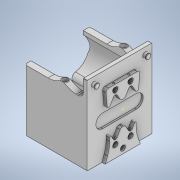
# Autodesk Inventor part: akkum_base2
Saved by Autodesk Inventor 2022 (Build 260153000, 153)
## iProperties
Created: 2024-07-26
Part Number: akkum_base2
Material: Типовые
Document SubType Name: Modeling
Designer: Капустяник Андрей
Density: 1 g/cm^3
Appearance: По умолчанию
Author: Капустяник Андрей
Autodesk Inventor part; units mm, degrees
ref_plane "YZ Plane" through (0, 0, 0) normal (1, 0, 0) x (0, 1, 0)
ref_plane "XZ Plane" through (0, 0, 0) normal (0, 1, 0) x (-1, 0, 0)
ref_plane "XY Plane" through (0, 0, 0) normal (0, 0, 1) x (1, 0, 0)
sketch "Эскиз1" plane through (0, 0, 0) normal (1, 0, 0) x (0, 1, 0)
  circle A0 centre (3.5, 9.3) radius 9.5 projected
  circle A1 centre (3.5, -9.3) radius 9.5 projected
  circle A2 centre (-12.6081, 0) radius 9.5 projected
  line L0 (-24, -20) -> (24, -20) projected
  line L1 (-24, 20) -> (-24, -20) projected
  line L2 (24, 20) -> (-24, 20) projected
  line L3 (13, -19) -> (13, 19) projected
  line L4 (24, -20) -> (24, 20) projected
  line L5 (-23.5, 19.5) -> (-23.5, -19.5)
  line L6 (-23.5, -19.5) -> (23.5, -19.5)
  line L7 (23.5, -19.5) -> (23.5, 19.5)
  line L8 (23.5, 19.5) -> (-23.5, 19.5)
  line L9 (-23.2, 19.2) -> (-23.2, -19.2)
  line L10 (-23.2, -19.2) -> (23.2, -19.2)
  line L11 (23.2, -19.2) -> (23.2, 19.2)
  line L12 (23.2, 19.2) -> (-23.2, 19.2)
  line L13 (13, 19.2) -> (13, -19.2)
  circle A3 centre (-8.3458, 11.2175) radius 2.5
  circle A4 centre (-8.3458, -11.2175) radius 2.5
  circle A5 centre (11.0835, 0) radius 2.5
  point P0 (0, 0)
  point P1 (13, 9.3)
  point P2 (13, -9.3)
  point P3 (-5.5236, -6.3293)
  point P4 (-5.5236, 6.3293)
  point P5 (5.4391, 0)
  point P6 (-5.8779, -10.818)
  point P7 (-9.2338, -8.8805)
  point P8 (-9.2338, 8.8805)
  point P9 (-5.8779, 10.818)
  point P10 (9.5036, 1.9375)
  point P11 (9.5036, -1.9375)
  dimension "d2" = 0.5
  dimension "d3" = 0.3
  dimension "d4" = 5
  dimension "d5" = 5
  dimension "d6" = 5
  constraints: 18 end point, 6 tangent, 3 centre point, 3 point on line, 1 collinear, 6 other
  measures "d2" distance between parallel lines of L2 L8
  measures "d3" distance between parallel lines of L8 L12
  measures "d4" diameter of A3
  measures "d5" diameter of A4
  measures "d6" diameter of A5
extrude "Выдавливание1" add sketch "Эскиз1" along normal blind 34.5 contours L3 A5 A0 | A0 A3 A2 A4 A1 L3 L13 L10 L9 L12 | A3 | A5 L3 | A5 L3 A1 | A4 picked at (11.5482, -0.1832)
sketch "Эскиз2" plane through (34.5, 0, 0) normal (1, 0, 0) x (0, 0, -1)
  line L0 (19.2, -23.2) -> (19.2, 13) projected
  line L1 (19.2, 13) -> (9.3, 13) projected
  arc A0 (10.818, -5.8779) -> (9.3, 13) centre (9.3, 3.5) ccw projected
  arc A1 (10.818, -5.8779) -> (8.8805, -9.2338) centre (11.2175, -8.3458) ccw projected
  arc A2 (-8.8805, -9.2338) -> (8.8805, -9.2338) centre (0, -12.6081) ccw projected
  arc A3 (-8.8805, -9.2338) -> (-10.818, -5.8779) centre (-11.2175, -8.3458) ccw projected
  arc A4 (-9.3, 13) -> (-10.818, -5.8779) centre (-9.3, 3.5) ccw projected
  line L2 (-9.3, 13) -> (-19.2, 13) projected
  line L3 (-19.2, 13) -> (-19.2, -23.2) projected
  line L4 (-19.2, -23.2) -> (19.2, -23.2) projected
  circle A5 centre (-9.3, 3.5) radius 7.5
  circle A6 centre (9.3, 3.5) radius 7.5
  circle A7 centre (0, -12.6081) radius 7.5
  circle A8 centre (11.2175, -8.3458) radius 4.5
  circle A9 centre (-11.2175, -8.3458) radius 4.5
  arc A10 (-1.9375, 9.5036) -> (1.9375, 9.5036) centre (0, 11.0835) ccw projected
  circle A11 centre (0, 11.0835) radius 4.5
  arc A12 (-1.9375, 9.5036) -> (-9.3, 13) centre (-9.3, 3.5) ccw projected
  arc A13 (-1.9375, 9.5036) -> (1.9375, 9.5036) centre (0, 11.0835) ccw projected
  arc A14 (9.3, 13) -> (1.9375, 9.5036) centre (9.3, 3.5) ccw projected
  line L5 (9.3, 13) -> (-9.3, 13) projected
  point P0 (0, 0)
  point P1 (-9.3, 13)
  point P2 (9.3, 13)
  point P3 (-3.4875, 8.2397)
  point P4 (3.4875, 8.2397)
  point P5 (10.4985, -3.9036)
  point P6 (7.011, -9.9442)
  point P7 (-7.011, -9.9442)
  point P8 (-10.4985, -3.9036)
  dimension "d7" = 15
  dimension "d8" = 15
  dimension "d9" = 15
  constraints: 6 centre point, 6 coincident, 3 tangent
  measures "d7" diameter of A5
  measures "d8" diameter of A6
  measures "d9" diameter of A7
extrude "Выдавливание2" add sketch "Эскиз2" against normal blind 1.7 contours L4 L3 L2 A4 A9 A2 A8 A0 L1 L0 | A0 A8 A6 A11 A14 | A14 A11 L5 | A8 A2 A1 A0 | A0 A1 A2 A8 | A14 A10 A12 A11 L5 | A11 A12 A10 A14 | A12 A11 A5 A9 A4 | L5 A11 A12 | A9 A2 A3 A4 | A4 A3 A2 A9 | A2 A9 A7 A8
sketch "Эскиз3" plane through (34.5, 0, 0) normal (1, 0, 0) x (0, 0, -1)
  line L0 (-15.5, 15.5) -> (-15.5, 17.5) projected
  line L1 (15.5, 17.5) -> (15.5, 15.5) projected
  line L2 (-15.5, 15.5) -> (15.5, 15.5)
  line L3 (15.5, 15.5) -> (15.5, 2)
  line L4 (15.5, 2) -> (-15.5, 2)
  line L5 (-15.5, 2) -> (-15.5, 15.5)
  point P0 (0, 0)
  constraints: 8 end point, 2 parallel, 1 collinear, 1 horizontal, 1 perpendicular
extrude "Выдавливание3" cut sketch "Эскиз3" against normal blind 2
sketch "Эскиз4" plane through (34.5, 0, 0) normal (1, 0, 0) x (0, 0, -1)
  line L0 (15.5, 13) -> (15.5, 7.7202) projected
  arc A0 (10.4985, -3.9036) -> (15.5, 7.7202) centre (9.3, 3.5) ccw projected
  arc A1 (10.4985, -3.9036) -> (7.011, -9.9442) centre (11.2175, -8.3458) ccw projected
  arc A2 (-7.011, -9.9442) -> (7.011, -9.9442) centre (0, -12.6081) ccw projected
  arc A3 (-7.011, -9.9442) -> (-10.4985, -3.9036) centre (-11.2175, -8.3458) ccw projected
  arc A4 (-15.5, 7.7202) -> (-10.4985, -3.9036) centre (-9.3, 3.5) ccw projected
  line L1 (-15.5, 7.7202) -> (-15.5, 13) projected
  line L2 (-15.5, 13) -> (-19.2, 13) projected
  line L3 (-19.2, 13) -> (-19.2, -23.2) projected
  line L4 (-19.2, -23.2) -> (19.2, -23.2) projected
  line L5 (19.2, -23.2) -> (19.2, 13) projected
  line L6 (19.2, 13) -> (15.5, 13) projected
  line L7 (20, 24) -> (-20, 24) projected
  line L8 (-20, 24) -> (-20, -24) projected
  line L9 (20, -24) -> (20, 24) projected
  line L10 (-20, -24) -> (20, -24) projected
  line L11 (19.2, 23.2) -> (-19.2, 23.2)
  line L12 (-19.2, 23.2) -> (-19.2, -23.2)
  line L13 (-19.2, -23.2) -> (19.2, -23.2)
  line L14 (19.2, -23.2) -> (19.2, 23.2)
  point P0 (0, 0)
  point P1 (19.2, 4.494)
  dimension "d14" = 0.8
  constraints: 8 end point, 3 other
  measures "d14" distance between parallel lines of L9 L14
extrude "Выдавливание4" add sketch "Эскиз4" along normal blind 4.7 contours L6 L5 L4 L3 L2 L1 A4 A3 A2 A1 A0 L0 | L0 A0 A1 A2 A3 A4 L1 L2 L12 L11 L14 L6
sketch "Эскиз5" plane through (39.2, 0, 0) normal (1, 0, 0) x (0, 0, -1)
  line L0 (-19.5, 23.5) -> (-19.5, -23) projected
  line L1 (-20, 23.5) -> (-19.5, 23.5) projected
  line L2 (-20, -23) -> (-20, 23.5) projected
  arc A0 (-20, -23) -> (-19, -24) centre (-19, -23) ccw projected
  line L3 (-19, -23.5) -> (-19, -24) projected
  arc A1 (-19.5, -23) -> (-19, -23.5) centre (-19, -23) ccw projected
  arc A2 (19, -23.5) -> (19.5, -23) centre (19, -23) ccw projected
  line L4 (19, -24) -> (19, -23.5) projected
  arc A3 (19, -24) -> (20, -23) centre (19, -23) ccw projected
  line L5 (20, 23.5) -> (20, -23) projected
  line L6 (19.5, 23.5) -> (20, 23.5) projected
  line L7 (19.5, -23) -> (19.5, 23.5) projected
  line L8 (19.2, 23.2) -> (-19.2, 23.2) projected
  line L9 (-19.2, 23.2) -> (-19.2, -23.2) projected
  line L10 (-19.2, -23.2) -> (19.2, -23.2) projected
  line L11 (19.2, -23.2) -> (19.2, 23.2) projected
  circle A4 centre (-19, -23) radius 0.2
  circle A5 centre (19, -23) radius 0.2
  circle A6 centre (19, 23) radius 0.2
  line L12 (19.2, -23.2) -> (19.2, 23.2) projected
  circle A7 centre (-19, 23) radius 0.2
  line L13 (-19.2, 23.2) -> (-19.2, -23.2) projected
  line L14 (19.2, 23.2) -> (-19.2, 23.2) projected
  point P0 (0, 0)
  point P1 (-19, -23.2)
  point P2 (-19.2, -23)
  point P3 (19.2, -23)
  point P4 (19, -23.2)
  point P5 (19, 23.2)
  point P6 (19.2, 23)
  point P7 (-19.2, 23)
  point P8 (-19, 23.2)
  dimension "d17" = 0.4
  dimension "d18" = 0.4
  constraints: 6 tangent, 4 centre point, 2 coincident
  measures "d17" diameter of A6
  measures "d18" diameter of A7
extrude "Выдавливание5" cut sketch "Эскиз5" against normal blind 200 contours L11 A6 L8 | A7 L9 L8 | L11 L10 A5 | A4 L10 L9
sketch "Эскиз7" plane through (34.5, 0, 0) normal (-1, 0, 0) x (0, 0, 1)
  arc A0 (-19, 23.2) -> (-19.2, 23) centre (-19, 23) ccw projected
  line L0 (-19.2, 13) -> (-19.2, 23) projected
  line L1 (-19.2, 13) -> (-15.5, 13) projected
  line L2 (-15.5, 13) -> (-15.5, 7.7202) projected
  arc A1 (-15.5, 7.7202) -> (-10.4985, -3.9036) centre (-9.3, 3.5) ccw projected
  arc A2 (-7.011, -9.9442) -> (-10.4985, -3.9036) centre (-11.2175, -8.3458) ccw projected
  arc A3 (-7.011, -9.9442) -> (7.011, -9.9442) centre (0, -12.6081) ccw projected
  arc A4 (10.4985, -3.9036) -> (7.011, -9.9442) centre (11.2175, -8.3458) ccw projected
  arc A5 (10.4985, -3.9036) -> (15.5, 7.7202) centre (9.3, 3.5) ccw projected
  line L3 (15.5, 7.7202) -> (15.5, 13) projected
  line L4 (15.5, 13) -> (19.2, 13) projected
  line L5 (19.2, 23) -> (19.2, 13) projected
  arc A6 (19.2, 23) -> (19, 23.2) centre (19, 23) ccw projected
  line L6 (-19, 23.2) -> (19, 23.2) projected
  line L7 (15.5, 13) -> (19.2, 13) projected
  line L8 (-15.5, 13) -> (15.5, 13)
  point P0 (0, 0)
  constraints: 2 end point, 1 collinear
extrude "Выдавливание6" cut sketch "Эскиз7" against normal blind 0.5 contours L6 A6 L5 L4 L8 L1 L0 A0
sketch "Эскиз11" plane through (0, 0, 0) normal (-1, 0, 0) x (0, 0, 1)
  line L0 (15.5, 13) -> (-15.5, 13) projected
  line L1 (-15.5, 13) -> (-15.5, 7.7202) projected
  arc A0 (-15.5, 7.7202) -> (-10.4985, -3.9036) centre (-9.3, 3.5) ccw projected
  arc A1 (-7.011, -9.9442) -> (-10.4985, -3.9036) centre (-11.2175, -8.3458) ccw projected
  arc A2 (-7.011, -9.9442) -> (7.011, -9.9442) centre (0, -12.6081) ccw projected
  arc A3 (10.4985, -3.9036) -> (7.011, -9.9442) centre (11.2175, -8.3458) ccw projected
  arc A4 (10.4985, -3.9036) -> (15.5, 7.7202) centre (9.3, 3.5) ccw projected
  line L2 (15.5, 7.7202) -> (15.5, 13) projected
  point P0 (0, 0)
extrude "Выдавливание8" cut sketch "Эскиз11" against normal up to surface (34.5 mm away)
sketch "Эскиз12" plane through (0, 13, 19.2) normal (0, 1, 0) x (1, 0, 0)
  arc A0 (-32.5, 38.2) -> (-34.5, 36.2) centre (-32.5, 36.2) ccw projected
  line L0 (-34.5, 36.2) -> (-34.5, 35.7) projected
  arc A1 (-34.5, 35.7) -> (-33.5, 34.7) centre (-33.5, 35.7) ccw projected
  line L1 (-33.5, 34.7) -> (-33, 34.7) projected
  arc A2 (-32.5, 34.2) -> (-33, 34.7) centre (-33, 34.2) ccw projected
  line L2 (-32.5, 34.2) -> (-32.5, 23.2) projected
  arc A3 (-33, 22.7) -> (-32.5, 23.2) centre (-33, 23.2) ccw projected
  line L3 (-33, 22.7) -> (-33.5, 22.7) projected
  arc A4 (-33.5, 22.7) -> (-34.5, 21.7) centre (-33.5, 21.7) ccw projected
  line L4 (-34.5, 21.7) -> (-34.5, 16.7) projected
  arc A5 (-34.5, 16.7) -> (-33.5, 15.7) centre (-33.5, 16.7) ccw projected
  line L5 (-33.5, 15.7) -> (-33, 15.7) projected
  arc A6 (-32.5, 15.2) -> (-33, 15.7) centre (-33, 15.2) ccw projected
  line L6 (-32.5, 15.2) -> (-32.5, 4.2) projected
  arc A7 (-33, 3.7) -> (-32.5, 4.2) centre (-33, 4.2) ccw projected
  line L7 (-33, 3.7) -> (-33.5, 3.7) projected
  arc A8 (-33.5, 3.7) -> (-34.5, 2.7) centre (-33.5, 2.7) ccw projected
  line L8 (-34.5, 2.7) -> (-34.5, 2.2) projected
  arc A9 (-34.5, 2.2) -> (-32.5, 0.2) centre (-32.5, 2.2) ccw projected
  line L9 (-32.5, 0.2) -> (-24.6, 0.2) projected
  arc A10 (32.5, 0.2) -> (34.5, 2.2) centre (32.5, 2.2) ccw projected
  line L10 (34.5, 2.2) -> (34.5, 2.7) projected
  arc A11 (34.5, 2.7) -> (33.5, 3.7) centre (33.5, 2.7) ccw projected
  line L11 (33.5, 3.7) -> (33, 3.7) projected
  arc A12 (32.5, 4.2) -> (33, 3.7) centre (33, 4.2) ccw projected
  line L12 (32.5, 4.2) -> (32.5, 15.2) projected
  arc A13 (33, 15.7) -> (32.5, 15.2) centre (33, 15.2) ccw projected
  line L13 (33, 15.7) -> (33.5, 15.7) projected
  arc A14 (33.5, 15.7) -> (34.5, 16.7) centre (33.5, 16.7) ccw projected
  line L14 (34.5, 16.7) -> (34.5, 21.7) projected
  arc A15 (34.5, 21.7) -> (33.5, 22.7) centre (33.5, 21.7) ccw projected
  line L15 (33.5, 22.7) -> (33, 22.7) projected
  arc A16 (32.5, 23.2) -> (33, 22.7) centre (33, 23.2) ccw projected
  line L16 (32.5, 23.2) -> (32.5, 34.2) projected
  arc A17 (33, 34.7) -> (32.5, 34.2) centre (33, 34.2) ccw projected
  line L17 (33, 34.7) -> (33.5, 34.7) projected
  arc A18 (33.5, 34.7) -> (34.5, 35.7) centre (33.5, 35.7) ccw projected
  line L18 (34.5, 35.7) -> (34.5, 36.2) projected
  arc A19 (34.5, 36.2) -> (32.5, 38.2) centre (32.5, 36.2) ccw projected
  line L19 (32.5, 38.2) -> (24.6, 38.2) projected
  line L20 (0, 0) -> (35, 0) projected
  line L21 (32.5, 0) -> (32.5, 3.7)
  line L22 (34.5, 3.7) -> (0, 3.7) projected
  line L23 (0, 38.4) -> (35, 38.4) projected
  line L24 (32.5, 38.4) -> (32.5, 34.7)
  line L25 (0, 34.7) -> (34.5, 34.7) projected
  line L26 (32.5, 36.55) -> (22.5, 36.55)
  line L27 (32.5, 1.85) -> (22.5, 1.85)
  circle A20 centre (22.5, 1.85) radius 1.5
  circle A21 centre (22.5, 1.85) radius 2
  circle A22 centre (22.5, 36.55) radius 1.5
  circle A23 centre (22.5, 36.55) radius 2
  arc A24 (-21.4, 1.2) -> (-20.4, 0.2) centre (-20.4, 1.2) ccw projected
  line L28 (-20.4, 0.2) -> (1.7, 0.2) projected
  arc A25 (20.4, 0.2) -> (21.4, 1.2) centre (20.4, 1.2) ccw projected
  line L29 (21.4, 1.2) -> (21.4, 1.85) projected
  arc A26 (23.6, 1.85) -> (21.4, 1.85) centre (22.5, 1.85) ccw projected
  line L30 (23.6, 1.85) -> (23.6, 1.2) projected
  arc A27 (23.6, 1.2) -> (24.6, 0.2) centre (24.6, 1.2) ccw projected
  line L31 (24.6, 0.2) -> (32.5, 0.2) projected
  arc A28 (24.6, 38.2) -> (23.6, 37.2) centre (24.6, 37.2) ccw projected
  line L32 (23.6, 37.2) -> (23.6, 36.55) projected
  arc A29 (21.4, 36.55) -> (23.6, 36.55) centre (22.5, 36.55) ccw projected
  line L33 (21.4, 36.55) -> (21.4, 37.2) projected
  arc A30 (21.4, 37.2) -> (20.4, 38.2) centre (20.4, 37.2) ccw projected
  line L34 (20.4, 38.2) -> (-20.4, 38.2) projected
  arc A31 (-20.4, 38.2) -> (-21.4, 37.2) centre (-20.4, 37.2) ccw projected
  line L35 (-21.4, 37.2) -> (-21.4, 36.55) projected
  arc A32 (-23.6, 36.55) -> (-21.4, 36.55) centre (-22.5, 36.55) ccw projected
  line L36 (-23.6, 36.55) -> (-23.6, 37.2) projected
  arc A33 (-23.6, 37.2) -> (-24.6, 38.2) centre (-24.6, 37.2) ccw projected
  line L37 (-24.6, 38.2) -> (-32.5, 38.2) projected
  arc A34 (-24.6, 0.2) -> (-23.6, 1.2) centre (-24.6, 1.2) ccw projected
  line L38 (-23.6, 1.2) -> (-23.6, 1.85) projected
  arc A35 (-21.4, 1.85) -> (-23.6, 1.85) centre (-22.5, 1.85) ccw projected
  line L39 (-21.4, 1.85) -> (-21.4, 1.2) projected
  arc A36 (1.7, 0.2) -> (2, 0.5) centre (1.7, 0.5) ccw projected
  line L40 (2, 0.5) -> (2, 0.9) projected
  arc A37 (2.3, 1.2) -> (2, 0.9) centre (2.3, 0.9) ccw projected
  line L41 (2.3, 1.2) -> (13.7, 1.2) projected
  arc A38 (14, 0.9) -> (13.7, 1.2) centre (13.7, 0.9) ccw projected
  line L42 (14, 0.9) -> (14, 0.5) projected
  arc A39 (14, 0.5) -> (14.3, 0.2) centre (14.3, 0.5) ccw projected
  line L43 (14.3, 0.2) -> (20.4, 0.2) projected
  point P0 (0, 19.2)
  point P1 (23.6303, 38.2)
  point P2 (21.3697, 38.2)
  point P3 (21.7401, 34.7)
  point P4 (23.2599, 34.7)
  point P5 (23.2599, 3.7)
  point P6 (21.7401, 3.7)
  point P7 (21.3697, 0.2)
  point P8 (23.6303, 0.2)
  point P9 (23.2599, 0)
  point P10 (21.7401, 0)
  point P11 (23.2599, 38.4)
  point P12 (21.7401, 38.4)
  point P13 (23.9331, 37.9451)
  point P14 (21.0669, 37.9451)
  point P15 (23.9331, 0.4549)
  point P16 (21.0669, 0.4549)
  dimension "d36" = 10
  dimension "d37" = 10
  dimension "d38" = 3
  dimension "d39" = 4
  dimension "d40" = 3
  dimension "d41" = 4
  constraints: 8 end point, 4 centre point, 4 coincident, 4 point on line, 2 horizontal, 2 midpoint, 2 vertical
  measures "d36" distance of L26.start L26.end
  measures "d37" distance of L27.start L27.end
  measures "d38" diameter of A20
  measures "d39" diameter of A21
  measures "d40" diameter of A22
  measures "d41" diameter of A23
extrude "Выдавливание9" add sketch "Эскиз12" along normal blind 2.3 contours A30 A22 L26 A23 L25 | A23 L23 A28 A22 A30 | A28 A23 L26 A22 | A21 L27 A20 A25 L22 | A21 A27 A20 L27 | A21 L20 A25 A20 A27
chamfer "Фаска1" distance 2.3 angle 45 4 edges at (20.5, 13, 17.35) (24.5, 13, 17.35) (20.5, 13, -17.35) (24.5, 13, -17.35)
fillet "Сопряжение1" radius 10 4 edges at (18.2001, 13, -17.35) (26.7999, 13, -17.35) (26.7999, 13, 17.35) (18.2001, 13, 17.35)
sketch "Эскиз14" plane through (0, -23.2, -19) normal (0, -1, 0) x (1, 0, 0)
  line L0 (-25, 4) -> (25, 4)
  line L1 (25, 4) -> (25, 34)
  line L2 (25, 34) -> (-25, 34)
  line L3 (-25, 34) -> (-25, 4)
  line L4 (-25, 4) -> (25, 34) construction
  line L5 (25, 4) -> (-25, 34) construction
  line L6 (14, 34) -> (2, 34)
  line L7 (2, 38.2) -> (2, 38) projected
  line L8 (2, 38.2) -> (14, 38.2)
  line L9 (14, 38.2) -> (14, 34)
  line L10 (14, 34) -> (2, 34)
  line L11 (2, 34) -> (2, 38.2)
  line L12 (14, 38) -> (14, 38.2) projected
  point P0 (0, 19)
  dimension "d51" = 30
  constraints: 22 end point, 4 parallel, 2 horizontal, 2 midpoint, 2 perpendicular, 1 collinear, 1 point on line
  measures "d51" distance of L1.end L0.end
extrude "Выдавливание11" cut sketch "Эскиз14" against normal blind 0.8 contours L3 L2 L1 L0
fillet "Сопряжение4" radius 0.15 3 edges at (12.5, -23.2, 15) (25, -23.2, 0) (12.5, -23.2, -15)
fillet "Сопряжение5" radius 3 1 edges at (35, 13, 0)
sketch "Эскиз15" plane through (39.2, 0, 0) normal (1, 0, 0) x (0, 0, -1)
  point P0 (0, 0)
sketch "Эскиз16" plane through (0, -23, -19.2) normal (0, 0, -1) x (-1, 0, 0)
  line L0 (-39.5, 46) -> (-40, 46) projected
  arc A0 (-39, 46.5) -> (-39.5, 46) centre (-39, 46) ccw projected
  line L1 (-39, 47) -> (-39, 46.5) projected
  arc A1 (-39, 47) -> (-40, 46) centre (-39, 46) ccw projected
  line L2 (-35, 46) -> (-39.2, 46) projected
  circle A2 centre (-39, 46) radius 0.2
  line L3 (-35, 46) -> (-35, 46.2) projected
  line L4 (-35, 46.2) -> (-39.2, 46.2) projected
  line L5 (-39.2, 46) -> (-39.2, 46.2) projected
  line L6 (-35, 46) -> (-39.2, 46) projected
  line L7 (0, 36) -> (-14.3263, 36) projected
  line L8 (-23.2599, 38.3) -> (-21.7401, 38.3) projected
  line L9 (-30.6737, 36) -> (-32, 36) projected
  arc A3 (-35, 39) -> (-32, 36) centre (-32, 39) ccw projected
  line L10 (-35, 39) -> (-35, 46) projected
  line L11 (-35, 46) -> (-39.2, 46) projected
  line L12 (-39.2, 0) -> (-39.2, 46) projected
  line L13 (0, 0) -> (-39.2, 0) projected
  line L14 (0, 0) -> (0, 36) projected
  line L15 (0, 0) -> (0, -0.2) projected
  line L16 (0, 0) -> (-39.2, 0) projected
  line L17 (-39.2, -0.2) -> (-39.2, 0) projected
  line L18 (0, -0.2) -> (-39.2, -0.2) projected
  line L19 (0, 0) -> (-39.2, 0) projected
  circle A4 centre (-39, 0) radius 0.2
  point P0 (0, 23)
  point P1 (-14.15, 0)
  point P2 (-39, -0.2)
  point P3 (-39, 46.2)
  constraints: 1 centre point, 1 coincident, 1 point on line, 1 tangent, 5 other
extrude "Выдавливание12" cut sketch "Эскиз16" against normal blind 50 contours L5 L4 A2 | A4 L18 L17
sketch "Эскиз17" plane through (39.2, 0, 0) normal (1, 0, 0) x (0, 0, -1)
  line L0 (-19, 23.2) -> (19, 23.2) projected
  line L1 (-19.2, 23) -> (-19.2, -23) projected
  line L2 (19.2, -23) -> (19.2, 23) projected
  arc A0 (-19.2, -23) -> (-19, -23.2) centre (-19, -23) ccw projected
  line L3 (-19, -23.2) -> (19, -23.2) projected
  arc A1 (19, -23.2) -> (19.2, -23) centre (19, -23) ccw projected
  arc A2 (19.2, 23) -> (19, 23.2) centre (19, 23) ccw projected
  arc A3 (-19, 23.2) -> (-19.2, 23) centre (-19, 23) ccw projected
  line L4 (-19.2, 23.2) -> (-15.2, 23.2)
  line L5 (19, 23.2) -> (-19, 23.2) projected
  line L6 (-19.2, 23.2) -> (-19.2, 19.2)
  line L7 (-19.2, 23) -> (-19.2, 16) projected
  line L8 (-19.2, 19.2) -> (-15.2, 19.2)
  line L9 (-15.2, 19.2) -> (-15.2, 23.2)
  circle A4 centre (-15.2, 19.2) radius 1.6
  circle A5 centre (-15.2, 19.2) radius 4
  circle A6 centre (-15.2, 19.2) radius 1.1
  line L10 (-15.2, 19.2) -> (-15.2, 15.2)
  line L11 (0, 23.2) -> (0, -23.2)
  circle A7 centre (15.2, 19.2) radius 1.1
  circle A8 centre (-15.2, 19.2) radius 4.25
  circle A9 centre (15.2, 19.2) radius 4.25
  line L12 (-15.2, 14.95) -> (15.2, 14.95)
  line L13 (-7, 12.95) -> (-6, 12.95)
  line L14 (-6, 12.95) -> (-6, -17.05)
  line L15 (-6, -17.05) -> (-7, -17.05)
  line L16 (-7, -17.05) -> (-7, 12.95)
  circle A10 centre (-10, -2.05) radius 3
  line L17 (-7, -2.05) -> (-10, -2.05)
  line L18 (7, 12.95) -> (6, 12.95)
  line L19 (6, 12.95) -> (6, -17.05)
  line L20 (6, -17.05) -> (7, -17.05)
  line L21 (7, -17.05) -> (7, 12.95)
  circle A11 centre (10, -2.05) radius 3
  line L22 (-15.2, 15.2) -> (-1.2, 15.2)
  circle A12 centre (-15.2, 19.2) radius 14.5602
  line L23 (-19.2, 19.2) -> (-19.2, -23.2)
  circle A13 centre (-15.2, 19.2) radius 42.4
  line L24 (-15.2, -23.2) -> (-20, -23.2)
  line L25 (-20, -23.2) -> (-20.5, -23.2)
  line L26 (-26.7027, -23) -> (-27.1951, -22.9132)
  line L27 (19, -24) -> (-19, -24) projected
  line L28 (-27.1951, -22.9132) -> (-25.4586, -13.0651)
  line L29 (-25.4586, -13.0651) -> (-24.9662, -13.1519)
  circle A14 centre (-15.2, 19.2) radius 33.7939
  circle A15 centre (-15.2, 19.2) radius 43.7396
  line L30 (-26.7027, -23) -> (-20, -23)
  line L31 (-20, -23) -> (-20, 23) projected
  line L32 (-25.4586, -13.0651) -> (-20, -13.0651)
  line L33 (-26.7027, -23) -> (-19.1392, 19.8946)
  line L34 (-26.4691, -21.675) -> (-18.5906, -23.0642)
  line L35 (-25.4586, -13.0651) -> (-15.2, -13.0651)
  line L36 (-15.2, -13.0651) -> (-15.2, -14.5939)
  line L37 (-15.2, 19.2) -> (-15.2, -14.5939)
  line L38 (-24.2716, -9.2127) -> (-19.2, -9.2127)
  line L39 (-24.9662, -13.1519) -> (-24.2716, -9.2127)
  line L40 (-11.2147, 18.8576) -> (-14.8281, -23.1984)
  line L41 (-11.2158, 19.5548) -> (-7.4714, -22.4897)
  circle A16 centre (-6.2798, -2.05) radius 3
  line L42 (-7, 12.95) -> (-7, 9.95)
  line L43 (-7, 9.95) -> (-6, 9.95)
  line L44 (-7, -17.05) -> (-7, -14.05)
  line L45 (-7, -14.05) -> (-6, -14.05)
  spline S0 degree 2 poles (-7, 9.95) (0.4395, -1.9931) (-7, -14.05) knots 0 0 0 1 1 1
  line L46 (-7, 9.95) -> (-8.0386, 11.6717)
  line L47 (-8.0386, 11.6717) -> (-7.1824, 12.1882)
  line L48 (-7.1824, 12.1882) -> (-6, 9.95)
  line L49 (-3.2803, -1.9976) -> (-2.2803, -1.9976)
  spline S1 degree 2 poles (-6, 9.95) (1.4395, -1.9931) (-6, -14.05) knots 0 0 0 1 1 1
  line L50 (-7, -14.05) -> (-8.0477, -15.7629)
  line L51 (-8.0477, -15.7629) -> (-7.1947, -16.2847)
  line L52 (-7.1947, -16.2847) -> (-6, -14.05)
  line L53 (-6.5, 9.95) -> (-7.6135, 11.9281)
  line L54 (-6.5, -14.05) -> (-7.6212, -16.0238)
  line L55 (-24.2716, -9.2127) -> (-20, -9.2127)
  circle A17 centre (-15.2, 19.2) radius 29.8258
  line L56 (-24.2716, -9.2127) -> (-15.2, -9.2127)
  line L57 (-15.2, -9.2127) -> (-15.2, -10.6258)
  line L58 (-14.5054, 23.1392) -> (-0.7181, 20.7082)
  point P0 (0, 0)
  dimension "d83" = 6
  dimension "d60" = 4
  dimension "d61" = 4
  dimension "d62" = 3.2
  dimension "d63" = 8
  dimension "d64" = 2.2
  dimension "d65" = 0.25
  dimension "d66" = 1
  dimension "d67" = 30
  dimension "d68" = 6
  dimension "d69" = 2
  dimension "d70" = 6
  dimension "d71" = 14
  dimension "d73" = 0.5
  dimension "d75" = 0.5
  dimension "d76" = 10
  dimension "d77" = 1
  dimension "d78" = 10
  dimension "d79" = 1.5288
  dimension "d80" = 4
  dimension "d82" = 10
  dimension "d84" = 3
  dimension "d85" = 3
  dimension "d87" = 1
  dimension "d88" = 1
  dimension "d90" = 1
  dimension "d91" = 2.27
  dimension "d92" = 2.27
  dimension "d93" = 4.2716
  dimension "d94" = 1.4131
  dimension "d95" = 10
  constraints: 102 end point, 23 point on line, 17 point on circle, 12 horizontal, 10 centre point, 10 perpendicular, 9 coincident, 9 tangent, 7 symmetric about line, 6 midpoint, 3 parallel, 3 vertical, 2 vertical alignment, 1 collinear, 19 other
  measures "d60" distance of L4.start L4.end
  measures "d61" distance of L4.start L6.end
  measures "d62" diameter of A4
  measures "d63" diameter of A5
  measures "d64" diameter of A6
  measures "d66" distance of L14.end L15.end
  measures "d67" distance of L13.end L14.end
  measures "d68" diameter of A10
  measures "d69" distance between parallel lines of L12 L13
  measures "d70" distance between parallel lines of L11 L14
  measures "d71" distance of L10.end L22.end
  measures "d73" distance of L24.end L25.end
  measures "d75" distance of L26.start L26.end
  measures "d76" distance of L26.end L28.end
  measures "d77" distance between parallel lines of L30 L27
  measures "d78" angle of L1 L33
  measures "d79" distance of L35.end L36.end
  measures "d80" distance of L29.end L38.start
  measures "d82" angle of L41 L40
  measures "d84" distance of L13.start L42.end
  measures "d85" distance of L15.end L44.end
  measures "d87" distance of L46.end L47.end
  measures "d88" distance of L49.start L49.end
  measures "d90" distance of L50.end L51.end
  measures "d91" distance of L53.start L53.end
  measures "d92" distance of L54.end L54.start
  measures "d93" distance of L38.start L55.end
  measures "d94" distance of L56.end L57.end
  measures "d95" angle of L22 L58
sketch "Эскиз18" plane through (39.2, 0, 0) normal (1, 0, 0) x (0, 0, -1)
  line L0 (-11.2158, 19.5548) -> (-7.4714, -22.4897) projected
  line L1 (-15.2, 14.95) -> (15.2, 14.95) projected
  line L2 (-7.4714, -22.4897) -> (-7.3326, -24.0477)
  line L3 (-10.5185, 19.6169) -> (-6.7741, -22.4276)
  line L4 (-6.7741, -22.4276) -> (-6.6354, -23.9856)
  line L5 (-10.1029, 14.95) -> (-9.2158, 4.9894)
  line L6 (-9.2158, 4.9894) -> (0, 4.9894)
  line L7 (0, 4.9894) -> (0, 14.95)
  line L8 (15.2, 14.95) -> (-15.2, 14.95)
  line L9 (10.1029, 14.95) -> (9.2158, 4.9894)
  line L10 (9.2158, 4.9894) -> (0, 4.9894)
  line L11 (-19.2, -23) -> (19.2, -23) projected
  line L12 (19.2, -23) -> (19.2, 23) projected
  line L13 (-19.2, 23) -> (19.2, 23) projected
  line L14 (-19.2, 23) -> (-19.2, -23) projected
  line L15 (-19, 23.2) -> (19, 23.2) projected
  arc A0 (19.2, 23) -> (19, 23.2) centre (19, 23) ccw projected
  arc A1 (-19, 23.2) -> (-19.2, 23) centre (-19, 23) ccw projected
  arc A2 (-19.2, -23) -> (-19, -23.2) centre (-19, -23) ccw projected
  line L16 (-19, -23.2) -> (19, -23.2) projected
  arc A3 (19, -23.2) -> (19.2, -23) centre (19, -23) ccw projected
  line L17 (-7, -14.05) -> (-6, -14.05) projected
  circle A4 centre (-4.5, 9.95) radius 0.4
  line L18 (-4.1536, 10.15) -> (-1.1741, 4.9894)
  line L19 (-4.8464, 10.15) -> (-7.8259, 4.9894)
  line L20 (-4.8464, 9.75) -> (-7.8486, 14.95)
  line L21 (-4.1536, 9.75) -> (-1.1514, 14.95)
  line L22 (-2.0174, 13.45) -> (-6.9826, 13.45)
  line L23 (-7, 12.95) -> (-6, 12.95) projected
  line L24 (-3.2803, -1.9976) -> (-2.2803, -1.9976) projected
  line L25 (-4.1536, -14.1453) -> (-1.1741, -8.9847)
  line L26 (-4.8464, -14.1453) -> (-7.8259, -8.9847)
  line L27 (-4.8464, -13.7453) -> (-7.8486, -18.9453)
  line L28 (-4.1536, -13.7453) -> (-1.1514, -18.9453)
  line L29 (-2.0174, -17.4453) -> (-6.9826, -17.4453)
  line L30 (-4.8464, -14.1453) -> (-7.8464, -14.1453)
  line L31 (-4.8464, -14.1453) -> (-1.8464, -14.1453) construction
  line L32 (-7.8464, -8.9491) -> (-7.8464, -23.3793)
  line L33 (-19.2, -23) -> (19.2, -23) projected
  line L34 (-4.8464, -14.1453) -> (-7.8464, -8.9491)
  line L35 (4.1536, 10.15) -> (1.1741, 4.9894)
  line L36 (4.8464, 10.15) -> (7.8259, 4.9894)
  line L37 (4.8464, 9.75) -> (7.8486, 14.95)
  line L38 (4.1536, 9.75) -> (1.1514, 14.95)
  line L39 (2.0174, 13.45) -> (6.9826, 13.45)
  line L40 (4.8464, -13.7453) -> (7.8486, -18.9453)
  line L41 (2.0174, -17.4453) -> (6.9826, -17.4453)
  line L42 (4.1536, -13.7453) -> (1.1514, -18.9453)
  line L43 (4.1536, -14.1453) -> (1.1741, -8.9847)
  line L44 (4.8464, -14.1453) -> (7.8259, -8.9847)
  line L45 (7.8464, -8.9491) -> (7.8464, -23.3793)
  line L46 (4.8464, -14.1453) -> (7.8464, -8.9491)
  line L47 (-1.1741, -8.9847) -> (1.1741, -8.9847)
  line L48 (-19, -23.2) -> (19, -23.2) projected
  line L49 (-10.3942, -23.2) -> (-7.8464, -16.2)
  line L50 (-7.8464, -16.2) -> (7.8464, -16.2)
  line L51 (10.3942, -23.2) -> (7.8464, -16.2)
  circle A5 centre (-15.2, 19.2) radius 1.1 projected
  circle A6 centre (15.2, 19.2) radius 1.1 projected
  circle A7 centre (-15.2, 19.2) radius 1.45
  circle A8 centre (15.2, 19.2) radius 1.45
  line L52 (-7, 9.95) -> (-6, 9.95) projected
  line L53 (-6.5, 9.95) -> (0, 9.95)
  line L54 (-6, 12.95) -> (-6, -17.05) projected
  circle A9 centre (-4.5, -13.9453) radius 0.4
  point P0 (0, 0)
  point P1 (-7.4259, -23)
  point P2 (-7.4081, -23.2)
  point P3 (4.9619, -13.9453)
  point P4 (7.8464, -23)
  point P5 (-7.8464, -23)
  point P6 (-4.9619, -13.9453)
  point P7 (-4.0381, -13.9453)
  point P8 (4.0381, -13.9453)
  point P9 (-9.2972, 5.9031)
  point P10 (9.2972, 5.9031)
  point P11 (4.9619, 9.95)
  point P12 (4.0381, 9.95)
  point P13 (1.1741, 4.9894)
  point P14 (10.3942, -23.2)
  point P15 (-4.0381, 9.95)
  point P16 (-4.9619, 9.95)
  dimension "d96" = 0.7
  dimension "d97" = 10
  dimension "d100" = 0.8
  dimension "d101" = 60
  dimension "d102" = 60
  dimension "d103" = 60
  dimension "d104" = 60
  dimension "d105" = 0.5
  dimension "d106" = 3
  dimension "d107" = 180
  dimension "d108" = 7
  dimension "d109" = 20
  dimension "d114" = 2.9
  dimension "d115" = 2.9
  dimension "d135" = 4.5
  constraints: 80 end point, 38 symmetric about line, 27 point on line, 8 point on circle, 5 horizontal, 4 centre point, 4 collinear, 4 tangent, 2 coincident, 2 midpoint, 2 perpendicular, 1 other
  measures "d96" distance between parallel lines of L0 L3
  measures "d97" distance of L5.start L5.end
  measures "d100" diameter of A4
  measures "d101" angle of L6 L18
  measures "d102" angle of L6 L19
  measures "d103" angle of L1 L21
  measures "d104" angle of L1 L20
  measures "d105" distance between parallel lines of L23 L22
  measures "d106" distance of L30.start L30.end
  measures "d107" angle of L30 L31
  measures "d108" distance between parallel lines of L48 L50
  measures "d109" angle of L32 L49
  measures "d114" diameter of A7
  measures "d115" diameter of A8
  measures "d135" distance from line of L7 A4.centre
extrude "Выдавливание13" cut sketch "Эскиз18" against normal blind 2 contours L1 L3 L32 L49 L0 | L0 L49 L11 L14 L13 L12 L51 L45 L46 L44 L40 L50 L42 L43 L47 L25 L28 A9 L27 L26 L54 L6 L10 L9 L1 | L49 L16 A2 L11 | L6 L54 L26 L34 L32 L3 | L22 L21 L18 A4 L19 L20 L54 L23 | L19 L54 L6 | A1 L15 A0 L13 | L50 L28 L29 L27 | L27 L54 L50 | L23 L54 L20 | L54 L19 L20 A4 L21 L18 L6 | L27 L30 A9 L25 L28 L50 L54 | L53 A4 L18 | L21 A4 L53 | L53 A4 L20 | L19 A4 L53 | A3 L16 L51 L11 | L27 L26 L30 | L39 L37 L36 L10 L35 L38 | A4 L53 | A4 L53 | L27 A9 L26 | A9 | L25 A9 L28 | L50 L40 L41 L42
fillet "Сопряжение6" radius 1.5 6 edges at (38.2, 14.95, 10.1029) (38.2, 14.95, -10.1029) (38.2, 4.9894, 1.1741) (38.2, 4.9894, -1.1741) (38.2, -8.9847, 1.1741) (38.2, -8.9847, -1.1741)
fillet "Сопряжение7" radius 1.2 8 edges at (38.2, -17.4453, 6.9826) (38.2, -17.4453, 2.0174) (38.2, -17.4453, -2.0174) (38.2, -17.4453, -6.9826) (38.2, 13.45, 6.9826) (38.2, 13.45, 2.0174) (38.2, 13.45, -2.0174) (38.2, 13.45, -6.9826)
fillet "Сопряжение8" radius 20 2 edges at (38.2, -16.2, 7.8464) (38.2, -16.2, -7.8464)
fillet "Сопряжение9" radius 0.5 6 edges at (38.2, -8.9491, 7.8464) (38.2, -8.9491, -7.8464) (38.2, 4.9894, 9.2158) (38.2, 4.9894, 7.8259) (38.2, 4.9894, -9.2158) (38.2, 4.9894, -7.8259)
sketch "Эскиз19" plane through (39.2, 19.2, 15.2) normal (1, 0, 0) x (0, 0, -1)
  circle A0 centre (0, 0) radius 1.45 projected
  circle A1 centre (30.4, 0) radius 1.45 projected
  circle A2 centre (0, 0) radius 1.55
  circle A3 centre (30.4, 0) radius 1.55
  point P0 (15.2, -19.2)
  dimension "d116" = 3.1
  dimension "d117" = 3.1
  constraints: 2 centre point, 2 coincident
  measures "d116" diameter of A2
  measures "d117" diameter of A3
extrude "Выдавливание14" add sketch "Эскиз19" against normal blind 0.5 contours A0 | A1 | A2 | A3
fillet "Сопряжение10" radius 0.2 4 edges at (39.2, 19.2, 16.75) (38.7, 19.2, 16.75) (39.2, 19.2, -13.65) (38.7, 19.2, -13.65)
sketch "Эскиз20" plane through (39.2, 0, 0) normal (1, 0, 0) x (0, 0, -1)
  line L0 (9.2564, 5.4451) -> (9.9575, 13.3169) projected
  arc A0 (9.9575, 13.3169) -> (8.4634, 14.95) centre (8.4634, 13.45) ccw projected
  line L1 (8.4634, 14.95) -> (-8.4634, 14.95) projected
  arc A1 (-8.4634, 14.95) -> (-9.9575, 13.3169) centre (-8.4634, 13.45) ccw projected
  line L2 (-9.9575, 13.3169) -> (-9.2564, 5.4451) projected
  line L3 (-7.6815, 5.2394) -> (-4.9619, 9.95) projected
  line L4 (-4.9619, 9.95) -> (-5.9434, 11.65) projected
  arc A2 (-4.9041, 13.45) -> (-5.9434, 11.65) centre (-4.9041, 12.25) ccw projected
  line L5 (-4.9041, 13.45) -> (-4.0959, 13.45) projected
  arc A3 (-3.0566, 11.65) -> (-4.0959, 13.45) centre (-4.0959, 12.25) ccw projected
  line L6 (-3.0566, 11.65) -> (-4.0381, 9.95) projected
  line L7 (-4.0381, 9.95) -> (-1.6071, 5.7394) projected
  arc A4 (-1.6071, 5.7394) -> (-0.3081, 4.9894) centre (-0.3081, 6.4894) ccw projected
  line L8 (-0.3081, 4.9894) -> (0.3081, 4.9894) projected
  arc A5 (0.3081, 4.9894) -> (1.6071, 5.7394) centre (0.3081, 6.4894) ccw projected
  line L9 (1.6071, 5.7394) -> (4.0381, 9.95) projected
  line L10 (4.0381, 9.95) -> (3.0566, 11.65) projected
  arc A6 (4.0959, 13.45) -> (3.0566, 11.65) centre (4.0959, 12.25) ccw projected
  line L11 (4.0959, 13.45) -> (4.9041, 13.45) projected
  arc A7 (5.9434, 11.65) -> (4.9041, 13.45) centre (4.9041, 12.25) ccw projected
  line L12 (5.9434, 11.65) -> (4.9619, 9.95) projected
  line L13 (4.9619, 9.95) -> (7.6815, 5.2394) projected
  arc A8 (7.8464, -10.8152) -> (6.9134, -10.5652) centre (7.3464, -10.8152) ccw projected
  line L14 (6.9134, -10.5652) -> (4.9619, -13.9453) projected
  line L15 (4.9619, -13.9453) -> (5.9434, -15.6453) projected
  arc A9 (4.9041, -17.4453) -> (5.9434, -15.6453) centre (4.9041, -16.2453) ccw projected
  line L16 (4.9041, -17.4453) -> (4.0959, -17.4453) projected
  arc A10 (3.0566, -15.6453) -> (4.0959, -17.4453) centre (4.0959, -16.2453) ccw projected
  line L17 (3.0566, -15.6453) -> (4.0381, -13.9453) projected
  line L18 (4.0381, -13.9453) -> (1.6071, -9.7347) projected
  arc A11 (1.6071, -9.7347) -> (0.3081, -8.9847) centre (0.3081, -10.4847) ccw projected
  line L19 (0.3081, -8.9847) -> (-0.3081, -8.9847) projected
  arc A12 (-0.3081, -8.9847) -> (-1.6071, -9.7347) centre (-0.3081, -10.4847) ccw projected
  line L20 (-1.6071, -9.7347) -> (-4.0381, -13.9453) projected
  line L21 (-4.0381, -13.9453) -> (-3.0566, -15.6453) projected
  arc A13 (-4.0959, -17.4453) -> (-3.0566, -15.6453) centre (-4.0959, -16.2453) ccw projected
  line L22 (-4.0959, -17.4453) -> (-4.9041, -17.4453) projected
  arc A14 (-5.9434, -15.6453) -> (-4.9041, -17.4453) centre (-4.9041, -16.2453) ccw projected
  line L23 (-5.9434, -15.6453) -> (-4.9619, -13.9453) projected
  line L24 (-4.9619, -13.9453) -> (-6.9134, -10.5652) projected
  arc A15 (-6.9134, -10.5652) -> (-7.8464, -10.8152) centre (-7.3464, -10.8152) ccw projected
  line L25 (-7.8464, -10.8152) -> (-7.8464, -12.6735) projected
  arc A16 (-9.0526, -19.5139) -> (-7.8464, -12.6735) centre (-27.8464, -12.6735) ccw projected
  line L26 (-9.0526, -19.5139) -> (-10.3214, -23) projected
  line L27 (-10.3214, -23) -> (10.3214, -23) projected
  line L28 (10.3214, -23) -> (9.0526, -19.5139) projected
  arc A17 (7.8464, -12.6735) -> (9.0526, -19.5139) centre (27.8464, -12.6735) ccw projected
  line L29 (7.8464, -12.6735) -> (7.8464, -10.8152) projected
  line L30 (-6.0381, 9.95) -> (-6.0413, 9.95) projected
  line L31 (-6.9607, 9.95) -> (-6.0413, 9.95)
  line L32 (4.0381, 9.95) -> (3.0566, 11.65) projected
  line L33 (5.9434, 11.65) -> (4.9619, 9.95) projected
  line L34 (4.0381, 9.95) -> (4.9619, 9.95)
  line L35 (-4.9619, -13.9453) -> (-4.0381, -13.9453)
  line L36 (4.0381, -13.9453) -> (4.9619, -13.9453)
  line L37 (3.0566, -15.6453) -> (4.0381, -13.9453) projected
  line L38 (-4.0381, -13.9453) -> (4.0381, -13.9453)
  line L39 (-6.0413, 9.95) -> (4.0381, 9.95)
  line L40 (-8.5016, 9.45) -> (6.4984, 9.45)
  line L41 (6.4984, 9.45) -> (6.4984, 10.45)
  line L42 (6.4984, 10.45) -> (-8.5016, 10.45)
  line L43 (-8.5016, 10.45) -> (-8.5016, 9.45)
  line L44 (-8.5016, 9.45) -> (6.4984, 10.45) construction
  line L45 (6.4984, 9.45) -> (-8.5016, 10.45) construction
  line L46 (-7.5, -14.4453) -> (7.5, -14.4453)
  line L47 (7.5, -14.4453) -> (7.5, -13.4453)
  line L48 (7.5, -13.4453) -> (-7.5, -13.4453)
  line L49 (-7.5, -13.4453) -> (-7.5, -14.4453)
  line L50 (-7.5, -14.4453) -> (7.5, -13.4453) construction
  line L51 (7.5, -14.4453) -> (-7.5, -13.4453) construction
  line L52 (8.1145, 4.9894) -> (8.7584, 4.9894) projected
  line L53 (-8.7584, 4.9894) -> (-8.1145, 4.9894) projected
  arc A18 (7.6815, 5.2394) -> (8.1145, 4.9894) centre (8.1145, 5.4894) ccw projected
  arc A19 (8.7584, 4.9894) -> (9.2564, 5.4451) centre (8.7584, 5.4894) ccw projected
  arc A20 (-9.2564, 5.4451) -> (-8.7584, 4.9894) centre (-8.7584, 5.4894) ccw projected
  arc A21 (-8.1145, 4.9894) -> (-7.6815, 5.2394) centre (-8.1145, 5.4894) ccw projected
  point P0 (0, 0)
  point P1 (-1.0016, 9.95)
  point P2 (0, -13.9453)
  dimension "d121" = 15
  dimension "d122" = 1
  dimension "d123" = 15
  dimension "d124" = 1
  constraints: 36 end point, 6 midpoint, 4 parallel, 3 horizontal, 2 perpendicular, 1 collinear
  measures "d121" distance of L42.end L41.end
  measures "d122" distance of L41.end L40.end
  measures "d123" distance of L48.end L47.end
  measures "d124" distance of L47.end L46.end
extrude "Выдавливание15" add sketch "Эскиз20" against normal up to surface (2 mm away) contours L40 L9 L34 L13 | L13 L12 L42 L41 L40 | L34 L10 L42 L12 | L40 L7 L39 L9 | L39 L6 L42 L10 | L40 L3 L39 L7 | L39 L4 L42 L6 | L40 L43 L42 L4 L3 | L48 L47 L46 L15 L14 | L14 L36 L18 L48 | L15 L46 L17 L36 | L18 L38 L20 L48 | L17 L46 L21 L38 | L20 L35 L24 L48 | L21 L46 L23 L35 | L24 L23 L46 L49 L48
sketch "Эскиз21" plane through (0, 14.95, -19) normal (0, -1, 0) x (1, 0, 0)
  line L0 (37.2, 8.6058) -> (39, 8.6058) projected
  line L1 (39, 29.3942) -> (39, 8.6058) projected
  line L2 (39, 29.3942) -> (37.2, 29.3942) projected
  line L3 (37.2, 29.3942) -> (37.2, 38) projected
  line L4 (0, 38) -> (37.2, 38) projected
  line L5 (25.15, 34.15) -> (0, 34.15) projected
  line L6 (25.15, 3.85) -> (25.15, 34.15) projected
  line L7 (0, 3.85) -> (25.15, 3.85) projected
  line L8 (0, 3.85) -> (0, 0) projected
  line L9 (0, 0) -> (37.2, 0) projected
  line L10 (37.2, 0) -> (37.2, 8.6058) projected
  ellipse E0 centre (39, 8.6786) end of major axis (38.8, 8.6786) minor radius 0.0728 (39, 8.6058) -> (39.2, 8.6786) ccw projected
  line L11 (39.2, 29.3214) -> (39.2, 8.6786) projected
  ellipse E1 centre (39, 29.3214) end of major axis (39.2, 29.3214) minor radius 0.0728 (39.2, 29.3214) -> (39, 29.3942) ccw projected
  line L12 (39, 29.3942) -> (39, 8.6058) projected
  line L13 (37.2, 29.3942) -> (37.2, 8.6058)
  line L14 (37.2, 38) -> (37.2, 0) projected
  line L15 (37.2, 24.2506) -> (39.2, 24.2506) projected
  line L16 (37.2, 22.7494) -> (37.2, 24.2506) projected
  line L17 (39.2, 22.7494) -> (37.2, 22.7494) projected
  line L18 (39.2, 24.2506) -> (39.2, 22.7494) projected
  line L19 (32.8, 12.2825) -> (32.8, 8.5015) projected
  line L20 (39.2, 13.7494) -> (37.2, 13.7494) projected
  line L21 (39.2, 15.2506) -> (39.2, 13.7494) projected
  line L22 (37.2, 15.2506) -> (39.2, 15.2506) projected
  line L23 (37.2, 13.7494) -> (37.2, 15.2506) projected
  line L24 (39.2, 22.7494) -> (39.2, 24.2506) projected
  line L25 (37.2, 22.7494) -> (39.2, 24.2506)
  line L26 (37.2, 15.2506) -> (39.2, 13.7494)
  circle A0 centre (38.2, 23.5) radius 0.6
  circle A1 centre (38.2, 14.5) radius 0.6
  line L27 (0, 38) -> (0, 34.15) projected
  point P0 (0, 19)
  point P1 (32.8, 11.989)
  point P2 (39.2, 10.5008)
  point P3 (39.2, 27.5008)
  dimension "d127" = 1.2
  dimension "d128" = 1.2
  constraints: 6 end point, 2 centre point, 2 midpoint, 1 collinear, 2 other
  measures "d127" diameter of A0
  measures "d128" diameter of A1
extrude "Выдавливание16" cut sketch "Эскиз21" along normal up to surface (29.3953 mm away) contours A1 L26 | L26 A1 | A0 L25 | L25 A0
sketch "Эскиз22" plane through (37.2, 0, 0) normal (1, 0, 0) x (0, 0, -1)
  circle A0 centre (-10, -2.05) radius 3 projected
  circle A1 centre (-6.2798, -2.05) radius 3 projected
  circle A2 centre (-6.2798, -2.05) radius 4
  circle A3 centre (-10, -2.05) radius 4
  line L0 (-10, 1.95) -> (-6.2798, 1.95)
  line L1 (-10, -6.05) -> (-6.2798, -6.05)
  line L2 (-0.3081, 4.9894) -> (0.3081, 4.9894) projected
  line L3 (0, 4.9894) -> (0, -8.9847)
  line L4 (0.3081, -8.9847) -> (-0.3081, -8.9847) projected
  circle A4 centre (6.2798, -2.05) radius 4
  circle A5 centre (10, -2.05) radius 4
  line L5 (10, 1.95) -> (6.2798, 1.95)
  line L6 (10, -6.05) -> (6.2798, -6.05)
  line L7 (-6.2798, -6.05) -> (6.2798, -6.05)
  line L8 (6.2798, 1.95) -> (-6.2798, 1.95)
  point P0 (0, 0)
  dimension "d131" = 8
  dimension "d132" = 8
  constraints: 14 end point, 8 point on circle, 6 symmetric about line, 4 centre point, 3 tangent, 2 coincident, 2 midpoint, 1 horizontal, 2 other
  measures "d131" diameter of A2
  measures "d132" diameter of A3
extrude "Выдавливание17" cut sketch "Эскиз22" against normal blind 1
fillet "Сопряжение11" radius 1 16 edges at (38.2, -14.4453, 5.2506) (38.2, -14.4453, 3.7494) (38.2, -13.4453, 5.2506) (38.2, -13.4453, 3.7494) (38.2, -14.4453, -3.7494) (38.2, -13.4453, -3.7494) (38.2, -13.4453, -5.2506) (38.2, -14.4453, -5.2506) (38.2, 10.45, 5.2506) (38.2, 9.45, 5.2506) (38.2, 10.45, 3.7494) (38.2, 9.45, 3.7494) (38.2, 10.45, -3.7494) (38.2, 9.45, -3.7494) (38.2, 9.45, -5.2506) (38.2, 10.45, -5.2506)
fillet "Сопряжение12" radius 0.2 40 edges at (38.7936, 10.45, -4.4125) (38.7936, 10.45, -4.5875) (38.2, 10.5457, -5.1) (37.6, 10.45, -4.5) (38.2, 10.5457, -3.9) (37.6, 9.45, -4.5) (38.2, 9.3543, -5.1) (38.7936, 9.45, -4.5875) (38.7936, 9.45, -4.4125) (38.2, 9.3543, -3.9) (38.7936, 10.45, 4.4125) (38.7936, 10.45, 4.5875) (38.2, 10.5457, 3.9) (37.6, 10.45, 4.5) (38.2, 10.5457, 5.1) (37.6, 9.45, 4.5) (38.2, 9.3543, 3.9) (38.7936, 9.45, 4.5875) (38.7936, 9.45, 4.4125) (38.2, 9.3543, 5.1) (38.7936, -13.4453, 4.5875) (38.7936, -13.4453, 4.4125) (38.2, -13.3496, 3.9) (37.6, -13.4453, 4.5) (38.2, -13.3496, 5.1) (37.6, -14.4453, 4.5) (38.2, -14.5409, 3.9) (38.7936, -14.4453, 4.4125) (38.7936, -14.4453, 4.5875) (38.2, -14.5409, 5.1) (38.7936, -13.4453, -4.4125) (38.7936, -13.4453, -4.5875) (38.2, -13.3496, -5.1) (37.6, -13.4453, -4.5) (38.2, -13.3496, -3.9) (37.6, -14.4453, -4.5) (38.2, -14.5409, -5.1) (38.7936, -14.4453, -4.5875) (38.7936, -14.4453, -4.4125) (38.2, -14.5409, -3.9)
sketch "Эскиз23" plane through (39.2, 0, 0) normal (1, 0, 0) x (0, 0, -1)
  line L0 (-5.5392, -12.9453) -> (-6.9134, -10.5652) projected
  arc A0 (-6.9134, -10.5652) -> (-7.8464, -10.8152) centre (-7.3464, -10.8152) ccw projected
  line L1 (-7.8464, -10.8152) -> (-7.8464, -12.6735) projected
  arc A1 (-9.0526, -19.5139) -> (-7.8464, -12.6735) centre (-27.8464, -12.6735) ccw projected
  line L2 (-9.0526, -19.5139) -> (-10.3214, -23) projected
  line L3 (-10.3214, -23) -> (10.3214, -23) projected
  line L4 (10.3214, -23) -> (9.0526, -19.5139) projected
  arc A2 (7.8464, -12.6735) -> (9.0526, -19.5139) centre (27.8464, -12.6735) ccw projected
  line L5 (7.8464, -12.6735) -> (7.8464, -10.8152) projected
  arc A3 (7.8464, -10.8152) -> (6.9134, -10.5652) centre (7.3464, -10.8152) ccw projected
  line L6 (6.9134, -10.5652) -> (5.5392, -12.9453) projected
  arc A4 (4.6732, -13.4453) -> (5.5392, -12.9453) centre (4.6732, -12.4453) ccw projected
  line L7 (4.6732, -13.4453) -> (4.3268, -13.4453) projected
  arc A5 (3.4608, -12.9453) -> (4.3268, -13.4453) centre (4.3268, -12.4453) ccw projected
  line L8 (3.4608, -12.9453) -> (1.6071, -9.7347) projected
  arc A6 (1.6071, -9.7347) -> (0.3081, -8.9847) centre (0.3081, -10.4847) ccw projected
  line L9 (0.3081, -8.9847) -> (-0.3081, -8.9847) projected
  arc A7 (-0.3081, -8.9847) -> (-1.6071, -9.7347) centre (-0.3081, -10.4847) ccw projected
  line L10 (-1.6071, -9.7347) -> (-3.4608, -12.9453) projected
  arc A8 (-4.3268, -13.4453) -> (-3.4608, -12.9453) centre (-4.3268, -12.4453) ccw projected
  line L11 (-4.3268, -13.4453) -> (-4.6732, -13.4453) projected
  arc A9 (-5.5392, -12.9453) -> (-4.6732, -13.4453) centre (-4.6732, -12.4453) ccw projected
  line L12 (5.5392, -14.9453) -> (5.9434, -15.6453) projected
  arc A10 (4.9041, -17.4453) -> (5.9434, -15.6453) centre (4.9041, -16.2453) ccw projected
  line L13 (4.9041, -17.4453) -> (4.0959, -17.4453) projected
  arc A11 (3.0566, -15.6453) -> (4.0959, -17.4453) centre (4.0959, -16.2453) ccw projected
  line L14 (3.0566, -15.6453) -> (3.4608, -14.9453) projected
  arc A12 (4.3268, -14.4453) -> (3.4608, -14.9453) centre (4.3268, -15.4453) ccw projected
  line L15 (4.3268, -14.4453) -> (4.6732, -14.4453) projected
  arc A13 (5.5392, -14.9453) -> (4.6732, -14.4453) centre (4.6732, -15.4453) ccw projected
  line L16 (-4.6732, -14.4453) -> (-4.3268, -14.4453) projected
  arc A14 (-3.4608, -14.9453) -> (-4.3268, -14.4453) centre (-4.3268, -15.4453) ccw projected
  line L17 (-3.4608, -14.9453) -> (-3.0566, -15.6453) projected
  arc A15 (-4.0959, -17.4453) -> (-3.0566, -15.6453) centre (-4.0959, -16.2453) ccw projected
  line L18 (-4.0959, -17.4453) -> (-4.9041, -17.4453) projected
  arc A16 (-5.9434, -15.6453) -> (-4.9041, -17.4453) centre (-4.9041, -16.2453) ccw projected
  line L19 (-5.9434, -15.6453) -> (-5.5392, -14.9453) projected
  arc A17 (-4.6732, -14.4453) -> (-5.5392, -14.9453) centre (-4.6732, -15.4453) ccw projected
  line L20 (0.3081, -8.9847) -> (-0.3081, -8.9847) projected
  line L21 (0, -8.9847) -> (0, -23.05)
  line L22 (-15, -23.05) -> (15, -23.05) projected
  circle A18 centre (0, -20) radius 1.5
  line L23 (0, -20) -> (0, -23)
  line L24 (0, -23) -> (0, -8.9847)
  point P0 (0, 0)
  dimension "d139" = 3
  dimension "d142" = 3
  constraints: 6 end point, 3 midpoint, 1 centre point, 1 point on line, 1 vertical
  measures "d139" diameter of A18
  measures "d142" distance of L23.end L23.start
extrude "Выдавливание18" cut sketch "Эскиз23" against normal blind 3.5 contours A18 L21 | L21 A18
sketch "Эскиз24" plane through (0, 0, 0) normal (-1, 0, 0) x (0, 0, 1)
  arc A0 (-15.15, -23.2) -> (-15, -23.05) centre (-15.15, -23.05) ccw projected
  line L0 (-15, -23.05) -> (-15, -22.4) projected
  line L1 (-15, -22.4) -> (15, -22.4) projected
  line L2 (15, -22.4) -> (15, -23.05) projected
  arc A1 (15, -23.05) -> (15.15, -23.2) centre (15.15, -23.05) ccw projected
  line L3 (19, -23.2) -> (15.15, -23.2) projected
  arc A2 (19, -23.2) -> (19.2, -23) centre (19, -23) ccw projected
  line L4 (19.2, 13) -> (19.2, -23) projected
  line L5 (15.5, 13) -> (19.2, 13) projected
  line L6 (15.5, 13) -> (15.5, 10.6979) projected
  arc A3 (10.818, -5.8779) -> (15.5, 10.6979) centre (9.3, 3.5) ccw projected
  arc A4 (10.818, -5.8779) -> (8.8805, -9.2338) centre (11.2175, -8.3458) ccw projected
  arc A5 (-8.8805, -9.2338) -> (8.8805, -9.2338) centre (0, -12.6081) ccw projected
  arc A6 (-8.8805, -9.2338) -> (-10.818, -5.8779) centre (-11.2175, -8.3458) ccw projected
  arc A7 (-15.5, 10.6979) -> (-10.818, -5.8779) centre (-9.3, 3.5) ccw projected
  line L7 (-15.5, 10.6979) -> (-15.5, 13) projected
  line L8 (-19.2, 13) -> (-15.5, 13) projected
  line L9 (-19.2, -23) -> (-19.2, 13) projected
  arc A8 (-19.2, -23) -> (-19, -23.2) centre (-19, -23) ccw projected
  line L10 (-15.15, -23.2) -> (-19, -23.2) projected
  point P0 (0, 0)
extrude "Выдавливание19" cut sketch "Эскиз24" against normal blind 0.3
sketch "Эскиз25" plane through (22.5, 13, 17.35) normal (0, 1, 0) x (1, 0, 0)
  line L0 (-22.2, 36.55) -> (-8.1737, 36.55) projected
  line L1 (-22.2, 36.55) -> (-21.2, 36.55)
  line L2 (-21.2, 36.55) -> (-22.2, 35.55)
  line L3 (-22.2, 36.15) -> (-22.2, 28.168) projected
  line L4 (-22.2, 1.85) -> (-22.2, -1.85) projected
  line L5 (-22.2, 36.55) -> (-22.2, -1.85)
  line L6 (-22.2, -1.85) -> (-8.1737, -1.85) projected
  line L7 (-22.2, -1.85) -> (-22.2, -0.85)
  line L8 (-22.2, -0.85) -> (-21.2, -1.85)
  line L9 (-21.2, -1.85) -> (-22.2, -1.85)
  point P0 (-22.5, 17.35)
  point P1 (-22.2, 32.85)
  point P2 (-22.2, -0.85)
  dimension "d145" = 1
  dimension "d146" = 45
  dimension "d147" = 1
  constraints: 12 end point, 3 point on line, 1 collinear, 1 perpendicular
  measures "d145" distance of L0.start L1.end
  measures "d146" angle of L1 L2
  measures "d147" distance of L4.end L7.end
extrude "Выдавливание20" cut sketch "Эскиз25" against normal blind 50
sketch "Эскиз26" plane through (35, 16, 19.2) normal (0, 0, 1) x (1, 0, 0)
  line L0 (-9.85, -39.2) -> (-34.7, -39.2) projected
  line L1 (-34.7, -39.05) -> (-34.7, -38.4) projected
  line L2 (-34.7, -39.2) -> (-34.7, -38.4)
  line L3 (-34.7, -38.4) -> (-33.9, -39.2)
  point P0 (-35, -16)
  dimension "d150" = 0.8
  dimension "d151" = 45
  constraints: 4 end point, 1 collinear, 1 point on line
  measures "d150" distance of L0.end L1.end
  measures "d151" angle of L2 L3
extrude "Выдавливание21" cut sketch "Эскиз26" against normal blind 50
fillet "Сопряжение13" radius 0.5 2 edges at (0.7, -22.8, 18.6) (0.7, -22.8, -18.6)
